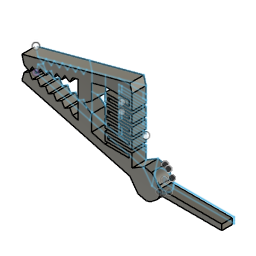
CompliantHands (Autodesk Fusion 360 design; units mm, degrees)
Autodesk Fusion 360 part; units mm, degrees
sketch "Sketch1" plane through (0, 0, 0) normal (0, 1, 0) x (1, 0, 0)
  line L0 (0, 0) -> (19.3185, 5.1764)
  line L1 (0, 0) -> (0.7765, -2.8978)
  line L2 (20.095, 2.2786) -> (19.3185, 5.1764)
  line L3 (0.7765, -2.8978) -> (3.6742, -2.1213)
  line L4 (3.6742, -2.1213) -> (6.572, -1.3449)
  line L5 (6.572, -1.3449) -> (9.4698, -0.5684)
  line L6 (9.4698, -0.5684) -> (12.3676, 0.2081)
  line L7 (12.3676, 0.2081) -> (15.2653, 0.9845)
  line L8 (15.2653, 0.9845) -> (18.1631, 1.761)
  line L9 (0.7765, -2.8978) -> (2.6136, -3.9584)
  line L10 (2.6136, -3.9584) -> (3.6742, -2.1213)
  line L11 (3.6742, -2.1213) -> (5.5114, -3.182)
  line L12 (5.5114, -3.182) -> (6.572, -1.3449)
  line L13 (6.572, -1.3449) -> (8.4091, -2.4055)
  line L14 (8.4091, -2.4055) -> (9.4698, -0.5684)
  line L15 (9.4698, -0.5684) -> (11.3069, -1.6291)
  line L16 (11.3069, -1.6291) -> (12.3676, 0.2081)
  line L17 (12.3676, 0.2081) -> (14.2047, -0.8526)
  line L18 (14.2047, -0.8526) -> (15.2653, 0.9845)
  line L19 (15.2653, 0.9845) -> (17.1025, -0.0762)
  line L20 (17.1025, -0.0762) -> (18.1631, 1.761)
  line L21 (20.095, 2.2786) -> (18.1631, 1.761)
  line L22 (12.3676, -8.3553) -> (15.2653, -9.1317)
  line L23 (9.4698, -7.5788) -> (12.3676, -8.3553)
  line L24 (9.4698, -7.5788) -> (11.3069, -6.5182)
  line L25 (8.4091, -5.7417) -> (9.4698, -7.5788)
  line L26 (6.572, -6.8024) -> (8.4091, -5.7417)
  line L27 (5.5114, -4.9653) -> (6.572, -6.8024)
  line L28 (3.6742, -6.0259) -> (5.5114, -4.9653)
  line L29 (0.7765, -5.2495) -> (2.6136, -4.1888)
  line L30 (2.6136, -4.1888) -> (3.6742, -6.0259)
  line L31 (11.3069, -6.5182) -> (12.3676, -8.3553)
  line L32 (12.3676, -8.3553) -> (14.2047, -7.2946)
  line L33 (14.2047, -7.2946) -> (15.2653, -9.1317)
  line L34 (15.2653, -9.1317) -> (17.1025, -8.0711)
  line L35 (15.2653, -9.1317) -> (18.1631, -9.9082)
  line L36 (17.1025, -8.0711) -> (18.1631, -9.9082)
  line L37 (0, -8.1472) -> (19.3185, -13.3236)
  line L38 (0, -8.1472) -> (0.7765, -5.2495)
  line L39 (0.7765, -5.2495) -> (3.6742, -6.0259)
  line L40 (6.572, -6.8024) -> (9.4698, -7.5788)
  line L41 (3.6742, -6.0259) -> (6.572, -6.8024)
  line L42 (20.095, -10.4258) -> (18.1631, -9.9082)
  line L43 (20.095, -10.4258) -> (19.3185, -13.3236)
  line L44 (20.095, 2.2786) -> (20.095, -10.4258)
  line L45 (19.3185, 5.1764) -> (38.637, 10.3528)
  line L46 (20.095, 2.2786) -> (39.4135, 7.455)
  line L47 (39.4135, 7.455) -> (38.637, 10.3528)
  line L48 (20.095, -10.4258) -> (39.4135, -15.6022)
  line L49 (19.3185, -13.3236) -> (38.637, -18.5)
  line L50 (38.637, -18.5) -> (39.4135, -15.6022)
  line L51 (20.095, 2.2786) -> (24.9246, 3.5727)
  line L52 (24.9246, 3.5727) -> (24.9246, -4.0736)
  line L53 (24.9246, -4.0736) -> (24.9246, -11.7199)
  line L54 (20.095, -4.0736) -> (22.095, -4.0736)
  line L55 (24.9246, -4.0736) -> (24.9246, -6.0736)
  line L56 (22.095, -4.0736) -> (24.9246, -6.0736)
  line L57 (24.9246, -4.0736) -> (24.9246, -2.0736)
  line L58 (22.095, -4.0736) -> (24.9246, -2.0736)
  line L59 (39.4135, 7.455) -> (39.4135, 4.8668)
  line L60 (39.4135, 4.8668) -> (29.7542, 4.8668)
  line L61 (39.4135, -15.6022) -> (39.4135, -13.014)
  line L62 (39.4135, -13.014) -> (29.7542, -13.014)
  line L63 (39.4135, -0.1332) -> (39.4135, 0.8668)
  line L64 (29.7542, -1.1332) -> (29.7542, -2.1332)
  line L65 (39.4135, -4.1332) -> (39.4135, -3.1332)
  line L66 (39.4135, -4.1332) -> (39.4135, -5.1332)
  line L67 (39.4135, -5.1332) -> (29.7542, -5.1332)
  line L68 (29.7542, -5.1332) -> (29.7542, -7.1332)
  line L69 (29.7542, -7.1332) -> (39.4135, -7.1332)
  line L70 (39.4135, -7.1332) -> (39.4135, -6.1332)
  line L71 (30.7542, -5.1332) -> (30.7542, -7.1332)
  line L72 (39.4135, -6.1332) -> (30.7542, -6.1332)
  line L73 (39.4135, -7.1332) -> (39.4135, -9.1332)
  line L74 (39.4135, -9.1332) -> (38.4135, -9.1332)
  line L75 (38.4135, -9.1332) -> (38.4135, -7.1332)
  line L76 (38.4135, -9.1332) -> (29.7542, -9.1332)
  line L77 (29.7542, -9.1332) -> (29.7542, -8.1332)
  line L78 (29.7542, -8.1332) -> (38.4135, -8.1332)
  line L79 (29.7542, -9.1332) -> (29.7542, -11.1332)
  line L80 (29.7542, -11.1332) -> (30.7542, -11.1332)
  line L81 (30.7542, -11.1332) -> (30.7542, -9.1332)
  line L82 (30.7542, -11.1332) -> (39.4135, -11.1332)
  line L83 (39.4135, -11.1332) -> (39.4135, -10.1332)
  line L84 (39.4135, -10.1332) -> (30.7542, -10.1332)
  line L85 (39.4135, -11.1332) -> (39.4135, -13.014)
  line L86 (39.4135, -11.1332) -> (38.4135, -11.1332)
  line L87 (38.4135, -11.1332) -> (38.4135, -13.014)
  line L88 (39.4135, 7.455) -> (43.713, 4.9027)
  line L89 (38.637, 10.3528) -> (41.5877, 14.3893)
  line L90 (41.5877, 14.3893) -> (43.713, 4.9027)
  line L91 (29.7542, -5.1332) -> (29.7542, -4.1332)
  line L92 (29.7542, -4.1332) -> (39.4135, -4.1332)
  line L93 (39.4135, -3.1332) -> (38.4135, -3.1332)
  line L94 (38.4135, -3.1332) -> (38.4135, -5.1332)
  line L95 (39.4135, -3.1332) -> (39.4135, -2.1332)
  line L96 (39.4135, -2.1332) -> (29.7542, -2.1332)
  line L97 (38.4135, -3.1332) -> (29.7542, -3.1332)
  line L98 (29.7542, -3.1332) -> (29.7542, -2.1332)
  line L99 (29.7542, -1.1332) -> (30.7542, -1.1332)
  line L100 (30.7542, -1.1332) -> (30.7542, -3.1332)
  line L101 (29.7542, -1.1332) -> (29.7542, -0.1332)
  line L102 (29.7542, -0.1332) -> (39.4135, -0.1332)
  line L103 (30.7542, -1.1332) -> (39.4135, -1.1332)
  line L104 (39.4135, -1.1332) -> (39.4135, -0.1332)
  line L105 (39.4135, -1.1332) -> (38.4135, -1.1332)
  line L106 (39.4135, 0.8668) -> (38.4135, 0.8668)
  line L107 (38.4135, 0.8668) -> (38.4135, -1.1332)
  line L108 (39.4135, 0.8668) -> (39.4135, 1.8668)
  line L109 (39.4135, 1.8668) -> (29.7542, 1.8668)
  line L110 (29.7542, 1.8668) -> (29.7542, 0.8668)
  line L111 (29.7542, 0.8668) -> (38.4135, 0.8668)
  line L112 (29.7542, 1.8668) -> (29.7542, 3.8668)
  line L113 (29.7542, 3.8668) -> (30.7542, 3.8668)
  line L114 (30.7542, 3.8668) -> (30.7542, 1.8668)
  line L115 (30.7542, 3.8668) -> (39.4135, 3.8668)
  line L116 (39.4135, 3.8668) -> (39.4135, 5.0729)
  line L117 (30.7542, 2.8668) -> (39.4135, 2.8668)
  line L118 (39.4135, 2.8668) -> (39.4135, 3.8668)
  line L119 (39.4135, 2.8668) -> (38.4135, 2.8668)
  line L120 (38.4135, 2.8668) -> (38.4135, 4.8668)
  circle A0 centre (45.9703, 10.3897) radius 3.4023
  line L121 (46.28, 5.4777) -> (43.713, 4.9027)
  line L122 (41.5877, 14.3893) -> (44.1548, 14.9643)
  spline S0 degree 5 poles (47.6847, 13.3285) (47.6048, 13.4012) (47.4459, 13.5431) (47.2099, 13.746) (46.8999, 13.9959) (46.5209, 14.2717) (46.1512, 14.5071) (45.7919, 14.6983) (45.4434, 14.8421) (45.106, 14.9387) (44.7788, 14.9908) (44.5247, 14.9995) (44.3382, 14.9886) (44.2156, 14.9737) (44.1548, 14.9643) knots 0 0 0 0 0 0 0.1 0.2 0.3 0.4 0.5 0.6 0.7 0.8 0.9 1 1 1 1 1 1
  spline S1 degree 5 poles (48.7311, 8.4013) (48.6822, 8.304) (48.5842, 8.1125) (48.4374, 7.835) (48.2415, 7.4848) (47.9966, 7.0826) (47.7516, 6.7194) (47.5065, 6.3991) (47.2614, 6.1252) (47.0161, 5.8979) (46.7708, 5.7146) (46.5745, 5.6007) (46.4273, 5.5326) (46.3291, 5.4948) (46.28, 5.4777) knots 0 0 0 0 0 0 0.1 0.2 0.3 0.4 0.5 0.6 0.7 0.8 0.9 1 1 1 1 1 1
  circle A1 centre (45.9703, 10.3897) radius 3.3
  line L123 (45.9703, 10.3897) -> (45.9703, 9.3897)
  line L124 (45.9703, 9.3897) -> (70.9703, 9.3897)
  line L125 (70.9703, 9.3897) -> (70.9703, 10.3897)
  line L126 (45.9703, 10.3897) -> (45.9703, 11.3897)
  line L127 (45.9703, 11.3897) -> (70.9703, 11.3897)
  line L128 (70.9703, 11.3897) -> (70.9703, 10.3897)
  point P0 (45.6581, 14.7479)
  point P1 (47.3897, 6.2744)
  dimension "d1" = 20
  dimension "d2" = 3
  dimension "d3" = 3
  dimension "d4" = 3
  dimension "d5" = 3
  dimension "d6" = 3
  dimension "d7" = 3
  dimension "d8" = 3
  dimension "d15" = 20
  dimension "d16" = 3
  dimension "d17" = 3
  dimension "d18" = 3
  dimension "d19" = 3
  dimension "d20" = 3
  dimension "d21" = 3
  dimension "d22" = 3
  dimension "d23" = 20
  dimension "d24" = 20
  dimension "d25" = 20
  dimension "d26" = 20
  dimension "d27" = 5
  dimension "d28" = 2
  dimension "d29" = 2
  dimension "d30" = 2
  dimension "d40" = 1
  dimension "d41" = 1
  dimension "d42" = 2
  dimension "d43" = 1
  dimension "d44" = 2
  dimension "d45" = 1
  dimension "d46" = 1
  dimension "d47" = 2
  dimension "d48" = 1
  dimension "d49" = 1
  dimension "d50" = 1
  dimension "d51" = 5
  dimension "d52" = 5
  dimension "d53" = 1
  dimension "d54" = 1
  dimension "d55" = 1
  dimension "d56" = 1
  dimension "d57" = 1
  dimension "d58" = 1
  dimension "d59" = 1
  dimension "d60" = 2
  dimension "d61" = 1
  dimension "d62" = 1
  dimension "d67" = 6.6
  dimension "d68" = 25
  dimension "d69" = 1
  dimension "d70" = 1
  constraint coincident L0.start L1.start
  constraint perpendicular L0 L1
  constraint perpendicular L0 L2
  constraint perpendicular L1 L3
  constraint perpendicular L1 L4
  constraint perpendicular L2 L21
  constraint perpendicular L37 L38
  constraint perpendicular L37 L43
  constraint perpendicular L38 L39
  constraint perpendicular L38 L41
  constraint perpendicular L42 L43
  constraint vertical L44
  constraint perpendicular L2 L45
  constraint perpendicular L2 L46
  constraint perpendicular L43 L48
  constraint perpendicular L43 L49
  constraint perpendicular L48 L50
  constraint perpendicular L2 L51
  constraint parallel L44 L52
  constraint coincident L48 L53.end
  constraint parallel L52 L53
  constraint midpoint L44 L54.start
  constraint perpendicular L44 L54
  constraint parallel L53 L55
  constraint coincident L52 L57.end
  constraint parallel L57 L59
  constraint midpoint L46 L60.end
  constraint perpendicular L59 L60
  constraint perpendicular L60 L61
  constraint midpoint L48 L62.end
  constraint perpendicular L61 L62
  constraint perpendicular L69 L70
  constraint coincident L67 L71.start
  constraint coincident L69 L71.end
  constraint perpendicular L69 L71
  constraint perpendicular L70 L72
  constraint perpendicular L69 L73
  constraint perpendicular L73 L74
  constraint coincident L69 L75.end
  constraint perpendicular L69 L75
  constraint perpendicular L68 L76
  constraint perpendicular L69 L77
  constraint midpoint L75 L78.end
  constraint perpendicular L76 L79
  constraint perpendicular L77 L80
  constraint coincident L76 L81.end
  constraint perpendicular L76 L81
  constraint perpendicular L73 L82
  constraint perpendicular L74 L83
  constraint midpoint L81 L84.end
  constraint perpendicular L62 L85
  constraint perpendicular L85 L86
  constraint coincident L62 L87.end
  constraint perpendicular L62 L87
  constraint perpendicular L67 L91
  constraint perpendicular L66 L92
  constraint perpendicular L65 L93
  constraint coincident L67 L94.end
  constraint perpendicular L92 L94
  constraint perpendicular L93 L95
  constraint perpendicular L64 L96
  constraint perpendicular L64 L97
  constraint perpendicular L96 L98
  constraint perpendicular L64 L99
  constraint perpendicular L96 L100
  constraint perpendicular L99 L101
  constraint perpendicular L63 L102
  constraint perpendicular L63 L103
  constraint perpendicular L102 L104
  constraint perpendicular L104 L105
  constraint perpendicular L63 L106
  constraint perpendicular L103 L107
  constraint perpendicular L106 L108
  constraint perpendicular L101 L109
  constraint perpendicular L109 L110
  constraint perpendicular L107 L111
  constraint perpendicular L109 L112
  constraint perpendicular L110 L113
  constraint coincident L109 L114.end
  constraint perpendicular L109 L114
  constraint perpendicular L59 L115
  constraint coincident L59 L116.end
  constraint perpendicular L60 L116
  constraint midpoint L114 L117.start
  constraint perpendicular L114 L117
  constraint perpendicular L115 L118
  constraint perpendicular L118 L119
  constraint coincident L60 L120.end
  constraint perpendicular L60 L120
  constraint coincident A0 S1.start
  constraint coincident A0 S0.start
  constraint perpendicular L90 L121
  constraint concentric A0 A1
  constraint coincident A0.centre A1.centre
  constraint perpendicular L123 L124
  constraint perpendicular L125 L127
  measures "d1" distance of L0.start L0.end
  measures "d2" distance of L0.start L1.end
  measures "d3" distance of L1.end L3.end
  measures "d4" distance of L3.end L4.end
  measures "d5" distance of L4.end L5.end
  measures "d6" distance of L5.end L6.end
  measures "d7" distance of L6.end L7.end
  measures "d8" distance of L7.end L8.end
  measures "d15" distance of L37.start L37.end
  measures "d16" distance of L37.start L29.start
  measures "d17" distance of L29.start L28.start
  measures "d18" distance of L28.start L26.start
  measures "d19" distance of L23.start L26.start
  measures "d20" distance of L22.start L23.start
  measures "d21" distance of L22.end L22.start
  measures "d22" distance of L22.end L35.end
  measures "d23" distance of L0.end L45.end
  measures "d24" distance of L2.start L46.end
  measures "d25" distance of L42.start L48.end
  measures "d26" distance of L37.end L49.end
  measures "d27" distance of L2.start L51.end
  measures "d28" distance of L54.start L54.end
  measures "d29" distance of L52.end L55.end
  measures "d30" distance of L52.end L57.end
  measures "d40" distance of L65.start L65.end
  measures "d41" distance of L65.start L66.end
  measures "d42" distance of L67.end L68.end
  measures "d43" distance of L69.end L70.end
  measures "d44" distance of L69.end L73.end
  measures "d45" distance of L73.end L74.end
  measures "d46" distance of L76.end L77.end
  measures "d47" distance of L76.end L79.end
  measures "d48" distance of L79.end L80.end
  measures "d49" distance of L82.end L83.end
  measures "d50" distance of L82.end L86.end
  measures "d51" distance of L46.end L88.end
  measures "d52" distance of L45.end L89.end
  measures "d53" distance of L67.end L91.end
  measures "d54" distance of L65.end L93.end
  measures "d55" distance of L65.end L95.end
  measures "d56" distance of L64.start L99.end
  measures "d57" distance of L64.start L101.end
  measures "d58" distance of L103.end L105.end
  measures "d59" distance of L63.end L108.end
  measures "d60" distance of L109.end L112.end
  measures "d61" distance of L112.end L113.end
  measures "d62" distance of L117.end L119.end
  measures "d67" diameter of A1
  measures "d68" distance of A0.centre L125.end
  measures "d69" distance of A0.centre L123.end
  measures "d70" distance of A0.centre L126.end
extrude "Extrude1" add sketch "Sketch1" against normal blind 5 contours L0 L1 L2 L3 L4 L5 L6 L7 L8 L21 | L2 L45 L46 L47 L51 | L3 L9 L10 | L44 L46 L51 L52 L54 L58 | L4 L11 L12 | L8 L19 L20 | L44 L48 L53 L54 L56 | L46 L59 L60 L116 | L5 L13 L14 | L7 L17 L18 | L22 L23 L35 L37 L38 L39 L40 L41 L42 L43 | L43 L48 L49 L50 | L6 L15 L16 | L34 L35 L36 | L60 L115 L116 L120 | L22 L32 L33 | L48 L61 L62 | L114 L115 L117 L120 | L115 L117 L118 L119 L120 | L23 L24 L31 | L29 L30 L39 | L62 L82 L85 L86 L87 | L109 L112 L113 L114 | L25 L26 L40 | L27 L28 L41 | L81 L82 L83 L84 L86 | L76 L79 L80 L81 | L106 L108 L109 L110 L111 | L75 L76 L77 L78 | L63 L102 L106 L107 | L69 L73 L74 L75 | L99 L101 L102 L103 L107 | L102 L103 L104 L105 L107 | L69 L70 L71 L72 | L64 L96 L99 L100 | L67 L68 L69 L71 | L96 L97 L98 L100 | L93 L95 L96 L97 L100 | L67 L91 L92 L94 | L65 L92 L93 L94 | L66 L67 L92 L94 makes body 1
extrude "Extrude2" add sketch "Sketch1" against normal blind 5 contours L47 L88 L89 L90 | L90 A0 L122 S0 | L90 A0 L121 S1 bodies 1
extrude "Extrude3" add sketch "Sketch1" against normal blind 0.5 contours A0 A1 L124 L127 | A0 A1 L124 L127 | A1 L123 L124 L126 L127 | A1 L123 L124 L126 L127 bodies 1
extrude "Extrude4" add sketch "Sketch1" along normal blind -5 and the other way blind 4.5 contours A0 A1 L124 L127 | A0 A1 L124 L127 | A1 L123 L124 L126 L127 | A1 L123 L124 L126 L127 bodies 1
extrude "Extrude5" add sketch "Sketch1" along normal blind -4.4 and the other way blind 0.6 separate body contours A0 L124 L125 L127 L128 | A0 A1 L124 L127 | A1 L123 L124 L126 L127 | A1 L123 L124 L126 L127 picked at (49.1795, 11.2806) makes body 2
